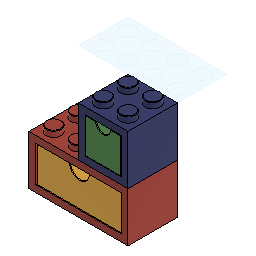
Lego Desktop Organizer (Drawer) (Autodesk Fusion 360 design; units mm, degrees)
Autodesk Fusion 360 part; units mm, degrees
note: some values were not read from the file. Set by a fixed rule: which face or edge a step refers to.
sketch "Sketch1" plane through (0, 0, 0) normal (0, 0, 1) x (1, 0, 0)
  line L0 (0, 0) -> (200, 0)
  line L1 (200, 0) -> (200, 100)
  line L2 (200, 100) -> (0, 100)
  line L3 (0, 100) -> (0, 0)
  dimension "d1" = 200
  dimension "d2" = 100
  constraint horizontal L0
  constraint vertical L1
  constraint horizontal L2
  constraint vertical L3
  constraint coincident L0.start L3.end
  measures "d1" distance of L0.start L0.end
  measures "d2" distance of L0.start L2.end
extrude "Extrude1" add sketch "Sketch1" along normal blind 100 makes body 1
sketch "Sketch3" plane through (0, 0, 100) normal (0, 0, 1) x (-1, 0, 0)
  line L0 (0, -100) -> (0, 0)
  line L1 (0, 0) -> (-200, 0)
  line L2 (-200, 0) -> (-200, -100)
  line L3 (-200, -100) -> (0, -100)
  circle A0 centre (-25, -75) radius 15
  dimension "d13" = 30
  dimension "d14" = 25
  dimension "d15" = 25
  measures "d13" diameter of A0
  measures "d14" distance of L3 A0.centre
  measures "d15" distance of L0 A0.centre
extrude "Extrude3" add sketch "Sketch3" along normal blind 12 contours A0 bodies 1
pattern_linear "R-Pattern2" count 4 spacing 50 along (1, 0, 0) count 2 spacing 50 along (0, -1, 0) of "Extrude3"
shell "Shell3" thickness 14 removed faces 1 at (66.6667, 0, 33.3333) on bodies 1
sketch "Sketch8" plane through (0, 0, 14) normal (0, 0, 1) x (-1, 0, 0)
  line L0 (-14, -86) -> (-14, 0)
  line L1 (-14, 0) -> (-186, 0)
  line L2 (-186, 0) -> (-186, -86)
  line L3 (-186, -86) -> (-14, -86)
  line L4 (-36.2601, 44.0301) -> (-206.2601, 44.0301)
  line L5 (-206.2601, 44.0301) -> (-206.2601, 128.0301)
  line L6 (-206.2601, 128.0301) -> (-36.2601, 128.0301)
  line L7 (-36.2601, 128.0301) -> (-36.2601, 44.0301)
  dimension "d26" = 170
  dimension "d27" = 84
  constraint horizontal L4
  constraint vertical L5
  constraint horizontal L6
  constraint vertical L7
  measures "d26" distance of L4.start L4.end
  measures "d27" distance of L4.start L6.end
extrude "Extrude4" add sketch "Sketch8" along normal blind 70 separate body contours L4 L5 L6 L7 makes body 2
shell "Shell5" thickness 2 removed faces 1 at (92.9267, -72.0301, 84) on bodies 2
hole "Hole1" at (121.2601, -128.0301, 84) direction (0, 1, 0) diameter 40 depth 45 tip angle 118 bodies 2
extrude "Extrude5" add 1 faces at (93.5934, -72.6967, 16) along direction (0, 0, 1) blind 2 on bodies 2 bodies 2
sketch "Sketch10" plane through (0, 0, 0) normal (0, 0, 1) x (1, 0, 0)
  line L0 (10, 10) -> (190, 10)
  line L1 (190, 10) -> (190, 90)
  line L2 (190, 90) -> (10, 90)
  line L3 (10, 90) -> (10, 10)
  dimension "d38" = 180
  dimension "d39" = 80
  constraint horizontal L0
  constraint vertical L1
  constraint horizontal L2
  constraint vertical L3
  measures "d38" distance of L0.start L0.end
  measures "d39" distance of L0.start L2.end
sketch "Sketch11" plane through (0, 0, 100) normal (0, 0, 1) x (-1, 0, 0)
  circle A0 centre (-175, -25) radius 15
  circle A1 centre (-125, -25) radius 15
  circle A2 centre (-75, -25) radius 15
  circle A3 centre (-25, -25) radius 15
  circle A4 centre (-175, -75) radius 15
  circle A5 centre (-125, -75) radius 15
  circle A6 centre (-75, -75) radius 15
  circle A7 centre (-25, -75) radius 15
  line L0 (0, -100) -> (0, 0)
  line L1 (0, 0) -> (-200, 0)
  line L2 (-200, 0) -> (-200, -100)
  line L3 (-200, -100) -> (0, -100)
  line L4 (-175, -25) -> (-125, -75)
  constraint coincident A0.centre L4.start
  constraint coincident A5.centre L4.end
sketch "Sketch12" plane through (0, 0, 0) normal (0, 0, -1) x (1, 0, 0)
  line L0 (0, 0) -> (0, -100)
  line L1 (0, -100) -> (200, -100)
  line L2 (200, -100) -> (200, 0)
  line L3 (200, 0) -> (0, 0)
  line L4 (10, -10) -> (190, -10)
  line L5 (190, -10) -> (190, -90)
  line L6 (190, -90) -> (10, -90)
  line L7 (10, -90) -> (10, -10)
  dimension "d40" = 180
  dimension "d41" = 80
  constraint horizontal L4
  constraint vertical L5
  constraint horizontal L6
  constraint vertical L7
  measures "d40" distance of L4.start L4.end
  measures "d41" distance of L4.start L6.end
extrude "Extrude6" cut sketch "Sketch12" against normal blind 12 contours L4 L5 L6 L7 bodies 1
sketch "Sketch15" plane through (0, 0, 12) normal (0, 0, -1) x (1, 0, 0)
  line L0 (10, -90) -> (190, -90)
  line L1 (190, -90) -> (190, -10)
  line L2 (190, -10) -> (10, -10)
  line L3 (10, -10) -> (10, -90)
  circle A0 centre (50, -50) radius 15
  circle A1 centre (50, -50) radius 20
  circle A2 centre (150, -50) radius 15
  circle A3 centre (150, -50) radius 20
  dimension "d44" = 30
  dimension "d45" = 40
  dimension "d46" = 30
  dimension "d47" = 40
  constraint concentric A0 A1
  constraint concentric A2 A3
  measures "d44" diameter of A0
  measures "d45" diameter of A1
  measures "d46" diameter of A2
  measures "d47" diameter of A3
extrude "Extrude7" add sketch "Sketch15" along normal blind 12 contours A1 bodies 1
sketch "Sketch16" plane through (0, 0, 12) normal (0, 0, -1) x (1, 0, 0)
  line L0 (10, -90) -> (190, -90)
  line L1 (190, -90) -> (190, -10)
  line L2 (190, -10) -> (10, -10)
  line L3 (10, -10) -> (10, -90)
  circle A0 centre (50, -50) radius 20
  circle A1 centre (150, -50) radius 15
  circle A2 centre (150, -50) radius 20
  dimension "d50" = 30
  dimension "d51" = 40
  constraint concentric A1 A2
  measures "d50" diameter of A1
  measures "d51" diameter of A2
extrude "Extrude8" add sketch "Sketch16" along normal blind 12 contours A2 bodies 1
sketch "Sketch17" plane through (0, 0, 100) normal (0, 0, 1) x (-1, 0, 0)
  circle A0 centre (-175, -25) radius 15
  circle A1 centre (-125, -25) radius 15
  circle A2 centre (-75, -25) radius 15
  circle A3 centre (-25, -25) radius 15
  circle A4 centre (-175, -75) radius 15
  circle A5 centre (-125, -75) radius 15
  circle A6 centre (-75, -75) radius 15
  circle A7 centre (-25, -75) radius 15
  line L0 (0, -100) -> (0, 0)
  line L1 (0, 0) -> (-200, 0)
  line L2 (-200, 0) -> (-200, -100)
  line L3 (-200, -100) -> (0, -100)
sketch "Sketch18" plane through (0, 0, 12) normal (0, 0, -1) x (1, 0, 0)
  circle A0 centre (50, -50) radius 20
  line L0 (10, -90) -> (190, -90)
  line L1 (190, -90) -> (190, -10)
  line L2 (190, -10) -> (10, -10)
  line L3 (10, -10) -> (10, -90)
  circle A1 centre (150, -50) radius 20
  circle A2 centre (100, -50) radius 15
  circle A3 centre (100, -50) radius 20
  dimension "d54" = 30
  dimension "d55" = 40
  constraint concentric A2 A3
  measures "d54" diameter of A2
  measures "d55" diameter of A3
extrude "Extrude9" add sketch "Sketch18" along normal blind 12 contours A3 bodies 1
move_body "Move1" bodies 2 to x (1, 0, 0) y (0, 1, 0) z (0, 0, 1) at (-10, 0, 0)
move_body "Move2" bodies 2 to x (1, 0, 0) y (0, 1, 0) z (0, 0, 1) at (-10, 130, 0)
move_body "Move3" bodies 2 to x (1, 0, 0) y (0, 1, 0) z (0, 0, 1) at (0, -100, 0)
move_body "Move4" bodies 2 to x (1, 0, 0) y (0, 1, 0) z (0, 0, 1) at (-0.0001, 100, 0)
move_body "Move5" bodies 2 to x (1, 0, 0) y (0, 1, 0) z (0, 0, 1) at (-1, 0, 0)
fillet "Fillet2" radius 1 8 edges at (38.9849, 30.4242, 112) (38.9849, 80.4242, 112) (88.9849, 80.4242, 112) (88.9849, 30.4242, 112) (138.9849, 80.4242, 112) (138.9849, 30.4242, 112) (188.9849, 80.4242, 112) (188.9849, 30.4242, 112) on bodies 1
sketch "Sketch19" plane through (0, 0, 0) normal (0, 0, 1) x (1, 0, 0)
  line L0 (250, 100) -> (350, 100)
  line L1 (350, 100) -> (350, 0)
  line L2 (350, 0) -> (250, 0)
  line L3 (250, 0) -> (250, 100)
  dimension "d62" = 100
  dimension "d63" = 100
  constraint horizontal L0
  constraint vertical L1
  constraint horizontal L2
  constraint vertical L3
  measures "d62" distance of L0.start L0.end
  measures "d63" distance of L0.start L2.end
extrude "Extrude10" add sketch "Sketch19" along normal blind 100 separate body makes body 3
sketch "Sketch20" plane through (0, 0, 100) normal (0, 0, 1) x (-1, 0, 0)
  line L0 (-250, 0) -> (-350, 0)
  line L1 (-350, 0) -> (-350, -100)
  line L2 (-350, -100) -> (-250, -100)
  line L3 (-250, -100) -> (-250, 0)
  circle A0 centre (-275, -75) radius 15
  dimension "d66" = 30
  dimension "d67" = 25
  dimension "d68" = 25
  measures "d66" diameter of A0
  measures "d67" distance of L3 A0.centre
  measures "d68" distance of L2 A0.centre
extrude "Extrude11" add sketch "Sketch20" along normal blind 12 contours A0 bodies 3
pattern_linear "R-Pattern3" count 2 spacing 50 along (1, 0, 0) count 2 spacing 50 along (0, -1, 0) of "Extrude11"
shell "Shell6" thickness 14 removed faces 1 at (316.6667, 0, 33.3333) on bodies 3
sketch "Sketch21" plane through (0, 0, 0) normal (0, 0, -1) x (1, 0, 0)
  line L0 (350, 0) -> (250, 0)
  line L1 (250, 0) -> (250, -100)
  line L2 (250, -100) -> (350, -100)
  line L3 (350, -100) -> (350, 0)
  line L4 (260, -10) -> (340, -10)
  line L5 (340, -10) -> (340, -90)
  line L6 (340, -90) -> (260, -90)
  line L7 (260, -90) -> (260, -10)
  constraint horizontal L4
  constraint vertical L5
  constraint horizontal L6
  constraint vertical L7
extrude "Extrude12" cut sketch "Sketch21" against normal blind 12 contours L4 L5 L6 L7 bodies 3
sketch "Sketch22" plane through (0, 0, 12) normal (0, 0, -1) x (1, 0, 0)
  line L0 (260, -90) -> (340, -90)
  line L1 (340, -90) -> (340, -10)
  line L2 (340, -10) -> (260, -10)
  line L3 (260, -10) -> (260, -90)
  circle A0 centre (300, -50) radius 15
  circle A1 centre (300, -50) radius 20
  dimension "d78" = 30
  dimension "d79" = 40
  constraint concentric A0 A1
  measures "d78" diameter of A0
  measures "d79" diameter of A1
extrude "Extrude13" add sketch "Sketch22" along normal blind 12 contours A1 bodies 3
sketch "Sketch23" plane through (0, 0, 0) normal (0, 0, 1) x (1, 0, 0)
  line L0 (250, -20) -> (320, -20)
  line L1 (320, -20) -> (320, -90)
  line L2 (320, -90) -> (250, -90)
  line L3 (250, -90) -> (250, -20)
  dimension "d82" = 70
  dimension "d83" = 70
  constraint horizontal L0
  constraint vertical L1
  constraint horizontal L2
  constraint vertical L3
  measures "d82" distance of L0.start L0.end
  measures "d83" distance of L0.start L2.end
extrude "Extrude14" add sketch "Sketch23" along normal blind 70 separate body makes body 4
shell "Shell7" thickness 2 removed faces 1 at (273.3333, -43.3333, 70) on bodies 4
extrude "Extrude15" add 1 faces at (274, -44, 2) along direction (0, 0, 1) blind 2 on bodies 4 bodies 4
hole "Hole2" at (285, -90, 70) direction (0, 1, 0) diameter 30 depth 30 tip angle 118 bodies 4
move_body "Move9" bodies 4 to x (1, 0, 0) y (0, 1, 0) z (0, 0, 1) at (15, 0, 0)
move_body "Move10" bodies 4 to x (1, 0, 0) y (0, 1, 0) z (0, 0, 1) at (0, 90, 14.7)
move_body "Move11" bodies 4 3 to x (1, 0, 0) y (0, 1, 0) z (0, 0, 1) at (-150, 0, 100)
fillet "Fillet3" radius 1 4 edges at (138.9849, 30.4242, 212) (138.9849, 80.4242, 212) (188.9849, 80.4242, 212) (188.9849, 30.4242, 212) on bodies 3
move_body "Move13" bodies 1 2 3 4 to x (1, 0, 0) y (0, 0, -1) z (0, 1, 0) at (0, 0, 0)
move_body "Move14" bodies 1 2 3 4 to x (1, 0, 0) y (0, 0, 1) z (0, -1, 0) at (0, -100, -100)
named bodies: "2 x 4 Box", "2 x 4 Drawer", "2 x 2 Box", "2 x 2 Drawer"
